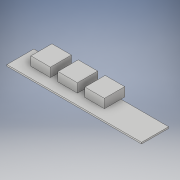
# Autodesk Inventor part: Usb ethernet hub
Saved by Autodesk Inventor 2018 (Build 220112000, 112)
## iProperties
Created: 2019-09-13
Part Number: Usb ethernet hub
Material: Generic
Document SubType Name: Modeling
Designer: Jacob
Density: 1 g/cm^3
Appearance: Default
Author: Jacob
Autodesk Inventor part; units mm, degrees
ref_plane "YZ Plane" through (0, 0, 0) normal (1, 0, 0) x (0, 1, 0)
ref_plane "XZ Plane" through (0, 0, 0) normal (0, 1, 0) x (-1, 0, 0)
ref_plane "XY Plane" through (0, 0, 0) normal (0, 0, 1) x (1, 0, 0)
sketch "Sketch1" plane through (0, 0, 0) normal (0, 1, 0) x (-1, 0, 0)
  line L0 (44.875, 9) -> (-44.875, 9)
  line L1 (-44.875, 9) -> (-44.875, -9)
  line L2 (-44.875, -9) -> (44.875, -9)
  line L3 (44.875, -9) -> (44.875, 9)
  line L4 (44.875, 9) -> (-44.875, -9) construction
  line L5 (-44.875, 9) -> (44.875, -9) construction
  point P0 (0, 0)
  dimension "d0" = 89.75
  dimension "d1" = 18
  constraints: 12 end point, 2 midpoint, 2 parallel, 1 horizontal, 1 perpendicular
  measures "d0" distance of L1.end L2.end
  measures "d1" distance of L0.end L1.end
extrude "Extrusion1" add sketch "Sketch1" along normal blind 1
sketch "Sketch2" plane through (0, 1, 0) normal (0, 1, 0) x (1, 0, 0)
  line L0 (44.875, -9) -> (44.875, 9) projected
  line L1 (44.875, 0) -> (-44.875, 0) construction
  line L2 (-44.875, 9) -> (-44.875, -9) projected
  line L3 (44.875, -7.15) -> (31.625, -7.15)
  line L4 (31.625, -7.15) -> (31.625, 7.15)
  line L5 (31.625, 7.15) -> (44.875, 7.15)
  line L6 (44.875, 7.15) -> (44.875, -7.15)
  line L7 (44.875, -7.15) -> (31.625, 7.15) construction
  line L8 (31.625, -7.15) -> (44.875, 7.15) construction
  point P0 (0, 0)
  point P1 (38.25, 0)
  dimension "d4" = 0
  dimension "d5" = 14.3
  dimension "d6" = 13.25
  constraints: 14 end point, 4 midpoint, 2 parallel, 1 horizontal, 1 perpendicular, 1 point on line
  measures "d4" distance between parallel lines of L0 L6
  measures "d5" distance of L3.end L4.end
  measures "d6" distance of L3.start L3.end
extrude "Extrusion2" [suppressed]
sketch "Sketch3" plane through (0, 0, 0) normal (0, -1, 0) x (1, 0, 0)
  line L0 (0, 0) -> (44.875, 0) construction
  line L1 (44.875, 9) -> (44.875, -9) projected
  line L2 (31.625, -7.15) -> (44.875, -7.15)
  line L3 (44.875, -7.15) -> (44.875, 7.15)
  line L4 (44.875, 7.15) -> (31.625, 7.15)
  line L5 (31.625, 7.15) -> (31.625, -7.15)
  line L6 (31.625, -7.15) -> (44.875, 7.15) construction
  line L7 (44.875, -7.15) -> (31.625, 7.15) construction
  point P0 (38.25, 0)
  dimension "d9" = 0
  dimension "d10" = 14.3
  dimension "d11" = 13.25
  constraints: 14 end point, 3 midpoint, 2 parallel, 1 horizontal, 1 perpendicular, 1 point on line
  measures "d9" distance between parallel lines of L1 L3
  measures "d10" distance of L4.end L2.start
  measures "d11" distance of L3.end L4.end
extrude "Extrusion3" [suppressed]
sketch "Sketch4" plane through (0, 1, 0) normal (0, 1, 0) x (1, 0, 0)
  line L0 (31.625, 7.15) -> (31.625, -7.15) projected
  line L1 (31.625, 0) -> (-44.875, 0) construction
  line L2 (-44.875, 9) -> (-44.875, -9) projected
  line L3 (-22.875, 12) -> (-35.875, 12)
  line L4 (-35.875, 12) -> (-35.875, -2)
  line L5 (-35.875, -2) -> (-22.875, -2)
  line L6 (-22.875, -2) -> (-22.875, 12)
  line L7 (-22.875, 12) -> (-35.875, -2) construction
  line L8 (-35.875, 12) -> (-22.875, -2) construction
  line L9 (44.875, 9) -> (-44.875, 9) projected
  line L10 (-44.875, -9) -> (44.875, -9) projected
  line L11 (-44.875, 4.75) -> (-18.375, 4.75) construction
  line L12 (-18.375, 4.75) -> (31.625, 4.75) construction
  line L13 (-4.875, 11.5) -> (-17.875, 11.5)
  line L14 (-17.875, 11.5) -> (-17.875, -2)
  line L15 (-17.875, -2) -> (-4.875, -2)
  line L16 (-4.875, -2) -> (-4.875, 11.5)
  line L17 (-4.875, 11.5) -> (-17.875, -2) construction
  line L18 (-17.875, 11.5) -> (-4.875, -2) construction
  line L19 (13.125, 11.5) -> (0.125, 11.5)
  line L20 (0.125, 11.5) -> (0.125, -2)
  line L21 (0.125, -2) -> (13.125, -2)
  line L22 (13.125, -2) -> (13.125, 11.5)
  line L23 (13.125, 11.5) -> (0.125, -2) construction
  line L24 (0.125, 11.5) -> (13.125, -2) construction
  point P0 (0, 0)
  point P1 (-11.375, 4.75)
  point P2 (6.625, 4.75)
  dimension "d14" = 22
  dimension "d15" = 13
  dimension "d17" = 3
  dimension "d18" = 7
  dimension "d19" = 13.5
  dimension "d20" = 13
  dimension "d21" = 5
  dimension "d22" = 5
  dimension "d23" = 13.5
  dimension "d24" = 13
  constraints: 42 end point, 7 midpoint, 7 parallel, 4 perpendicular, 3 horizontal, 3 point on line
  measures "d14" distance between parallel lines of L2 L6
  measures "d15" distance of L4.end L5.end
  measures "d17" distance between parallel lines of L9 L3
  measures "d18" distance between parallel lines of L10 L5
  measures "d19" distance of L15.end L13.start
  measures "d20" distance of L14.end L15.end
  measures "d21" distance between parallel lines of L6 L14
  measures "d22" distance between parallel lines of L16 L20
  measures "d23" distance of L21.end L19.start
  measures "d24" distance of L20.end L21.end
extrude "Extrusion4" add sketch "Sketch4" along normal blind 6
body "Solid1"
